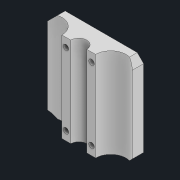
# Autodesk Inventor part: z-carriage-rear
Saved by Autodesk Inventor 2021 (Build 250183000, 183)
## iProperties
Created: 2021-06-07
Part Number: z-carriage-rear
Material: Generic
Document SubType Name: Modeling
Designer: arbra
Density: 1 g/cm^3
Appearance: Default
Author: arbra
Autodesk Inventor part; units mm, degrees
ref_plane "YZ Plane" through (0, 0, 0) normal (1, 0, 0) x (0, 1, 0)
ref_plane "XZ Plane" through (0, 0, 0) normal (0, 1, 0) x (-1, 0, 0)
ref_plane "XY Plane" through (0, 0, 0) normal (0, 0, 1) x (1, 0, 0)
sketch "Sketch1" plane through (0, 0, 0) normal (0, 1, 0) x (-1, 0, 0)
  line L0 (0, -16.8) -> (0, 2.8) construction
  line L1 (-37.1, 0) -> (37.1, 0) construction
  arc A0 (0, -5) -> (5, 0) centre (0, 0) ccw
  line L2 (5, 0) -> (10.5, 0)
  arc A1 (10.5, 0) -> (26.5, -6.9282) centre (20, 0) ccw
  line L3 (26.5, -6.9282) -> (26.5, -14)
  line L4 (26.5, -14) -> (0, -14)
  arc A2 (-5, 0) -> (0, -5) centre (0, 0) ccw
  line L5 (-5, 0) -> (-10.5, 0)
  arc A3 (-26.5, -6.9282) -> (-10.5, 0) centre (-20, 0) ccw
  line L6 (-26.5, -6.9282) -> (-26.5, -14)
  line L7 (-26.5, -14) -> (0, -14)
  dimension "d1" = 40
  dimension "d2" = 14
  dimension "d4" = 53
  dimension "d5" = 10
  dimension "d7" = 19
  constraints: 12 end point, 8 point on circle, 5 point on line, 5 symmetric about line, 4 centre point, 1 coincident, 1 perpendicular, 1 vertical, 2 other
  measures "d1" distance of A3.centre A1.centre
  measures "d2" distance between parallel lines of L4 L1
  measures "d4" distance between parallel lines of L3 L6
  measures "d5" diameter of A0
  measures "d7" diameter of A3
extrude "Extrusion1" add sketch "Sketch1" along normal mid plane 56
sketch "Sketch3" plane through (26.5, 28, -14) normal (0, 0, -1) x (-1, 0, 0)
  line L0 (26.5, -67.2) -> (26.5, 11.2) construction
  line L1 (-10.6, -28) -> (63.6, -28) construction
  line L2 (53, -56) -> (53, 0) projected
  point P0 (26.5, -28)
  point P1 (34.5, -5.5)
  point P2 (34.5, -50.5)
  point P3 (18.5, -5.5)
  point P4 (18.5, -50.5)
  dimension "d15" = 45
  dimension "d16" = 16
  constraints: 3 symmetric about line
  measures "d15" distance of point (34.5, -50.5) point (34.5, -5.5)
  measures "d16" distance of point (18.5, -5.5) point (34.5, -5.5)
hole "Hole1" at (-8, 22.5, -14) at (-8, -22.5, -14) at (8, 22.5, -14) at (8, -22.5, -14) direction (0, 0, 1) diameter 3.4 end through all counterbore diameter 6 counterbore depth 5
chamfer "Chamfer1" distance 4 angle 45 4 edges at (26.5, 28, -10.4641) (26.5, -28, -10.4641) (-26.5, -28, -10.4641) (-26.5, 28, -10.4641)
body "Solid1"
